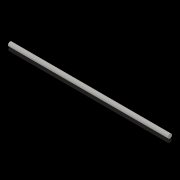
# Autodesk Inventor part: Shaft
Saved by Autodesk Inventor 2020 (Build 240168000, 168)
## iProperties
Created: 2020-08-26
Part Number: Shaft
Material: Steel
Document SubType Name: Modeling
Designer: alons
Density: 1 g/cm^3
Appearance: Steel
CustomPartVersion: 1
Author: alons
Length: 10.450 mm
Autodesk Inventor part; units mm, degrees
ref_plane "Start Plane" through (0, 0, 0) normal (1, 0, 0) x (0, 1, 0)
ref_plane "XZ Plane" through (0, 0, 0) normal (0, 1, 0) x (-1, 0, 0)
ref_plane "XY Plane" through (0, 0, 0) normal (0, 0, 1) x (1, 0, 0)
sketch "Main Sketch" plane through (0, 0, 0) normal (0, 0, 1) x (1, 0, 0)
  line L0 (0, 0) -> (10.45, 0)
  line L1 (0, 0) -> (0, 0.375)
  line L2 (0, 0.375) -> (0.25, 0.375)
  line L3 (4.5, 0.5) -> (5.5, 0.5)
  line L4 (5.5, 0.375) -> (5.7, 0.375)
  line L5 (5.7, 0.25) -> (7.7, 0.25)
  line L6 (7.7, 0.5) -> (8.2, 0.5)
  line L7 (9.7, 0.25) -> (10.2, 0.25)
  line L8 (10.45, 0.375) -> (10.45, 0)
  line L9 (10.2, 0.375) -> (10.45, 0.375)
  line L10 (10.2, 0.25) -> (10.2, 0.375)
  line L11 (7.7, 0.25) -> (7.7, 0.5)
  line L12 (8.2, 0.5) -> (8.2, 0.375)
  line L13 (5.5, 0.5) -> (5.5, 0.375)
  line L14 (5.7, 0.375) -> (5.7, 0.25)
  line L15 (2.5, 0.25) -> (2.5, 0.5)
  line L16 (2.5, 0.5) -> (3, 0.5)
  line L17 (0.25, 0.375) -> (0.25, 0.25)
  line L18 (0.25, 0.25) -> (2.5, 0.25)
  line L19 (8.2, 0.375) -> (9.2, 0.375)
  line L20 (9.2, 0.375) -> (9.2, 0.5)
  line L21 (9.7, 0.5) -> (9.7, 0.25)
  line L22 (9.2, 0.5) -> (9.7, 0.5)
  line L23 (3, 0.5) -> (3, 0.375)
  line L24 (3, 0.375) -> (4, 0.375)
  line L25 (4, 0.375) -> (4, 0.5)
  line L26 (4, 0.5) -> (4.5, 0.5)
  dimension "d3" = 0.75
  dimension "d4" = 1
  dimension "d5" = 0.75
  dimension "d6" = 0.5
  dimension "d7" = 1
  dimension "d8" = 0.5
  dimension "d9" = 0.75
  dimension "d13" = 1
  dimension "d14" = 0.5
  dimension "d15" = 0.75
  dimension "d16" = 1
  dimension "d17" = 0.75
  dimension "d18" = 1
  constraints: 54 end point, 13 vertical, 7 horizontal
  measures "d3" diameter of L2 L0
  measures "d4" diameter of L3 L0
  measures "d5" diameter of L4 L0
  measures "d6" diameter of L5 L0
  measures "d7" diameter of L6 L0
  measures "d8" diameter of L7 L0
  measures "d9" diameter of L9 L0
  measures "d13" diameter of L16 L0
  measures "d14" diameter of L18 L0
  measures "d15" diameter of L19 L0
  measures "d16" diameter of L22 L0
  measures "d17" diameter of L24 L0
  measures "d18" diameter of L26 L0
revolve "Revolution1" add sketch "Main Sketch" angle 360 about axis through (0, 0, 0) along (1, 0, 0)
fillet "Fillet2" [suppressed]
equation "\"Length\" = 10.45"
body "Solid1"
